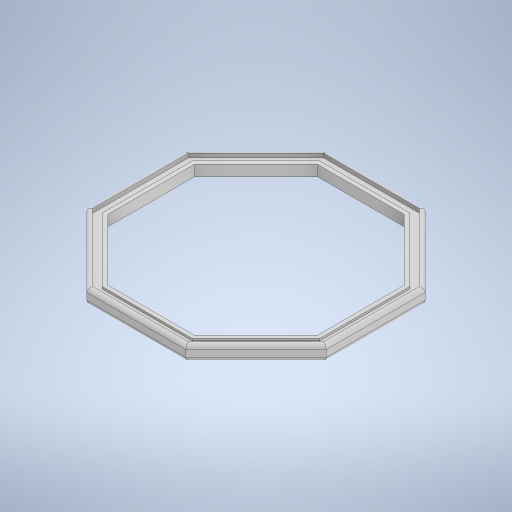
# Autodesk Inventor part: OV-PAM_ring_2
Saved by Autodesk Inventor 2024 (Build 280153000, 153)
## iProperties
Created: 2023-06-19
Part Number: OV-PAM_ring_2
Material: 일반
Document SubType Name: Modeling
Designer: jsw
Density: 1 g/cm^3
Appearance: 기본값
Author: jsw
Autodesk Inventor part; units mm, degrees
ref_plane "YZ Plane" through (0, 0, 0) normal (1, 0, 0) x (0, 1, 0)
sketch "스케치1" plane through (0, 0, 0) normal (0, 1, 0) x (-1, 0, 0)
  line L0 (-32.5919, 13.5) -> (-13.5, 32.5919)
  line L1 (-13.5, 32.5919) -> (13.5, 32.5919)
  line L2 (13.5, 32.5919) -> (32.5919, 13.5)
  line L3 (32.5919, 13.5) -> (32.5919, -13.5)
  line L4 (32.5919, -13.5) -> (13.5, -32.5919)
  line L5 (13.5, -32.5919) -> (-13.5, -32.5919)
  line L6 (-13.5, -32.5919) -> (-32.5919, -13.5)
  line L7 (-32.5919, -13.5) -> (-32.5919, 13.5)
  line L8 (35.5919, 14.7426) -> (35.5919, -14.7426)
  line L9 (35.5919, -14.7426) -> (14.7426, -35.5919)
  line L10 (14.7426, -35.5919) -> (-14.7426, -35.5919)
  line L11 (-14.7426, -35.5919) -> (-35.5919, -14.7426)
  line L12 (-35.5919, -14.7426) -> (-35.5919, 14.7426)
  line L13 (-35.5919, 14.7426) -> (-14.7426, 35.5919)
  line L14 (-14.7426, 35.5919) -> (14.7426, 35.5919)
  line L15 (14.7426, 35.5919) -> (35.5919, 14.7426)
  point P0 (0, 0)
  point P1 (0, 0)
  point P2 (0, 0)
  dimension "d0" = 27
  dimension "d1" = 3
  constraints: 32 end point, 2 coincident, 2 horizontal, 34 other
  measures "d0" distance of L2.end L3.end
  measures "d1" distance between parallel lines of L8 L3
extrude "돌출1" add sketch "스케치1" along normal blind 4.4 contours L0 L1 L2 L3 L4 L5 L6 L7 | L8 L9 L10 L11 L12 L13 L14 L15
sketch "스케치3" plane through (0, 0, 0) normal (0, -1, 0) x (1, 0, 0)
  line L0 (-13.5, 32.5919) -> (13.5, 32.5919)
  line L1 (13.5, 32.5919) -> (32.5919, 13.5)
  line L2 (32.5919, 13.5) -> (32.5919, -13.5)
  line L3 (32.5919, -13.5) -> (13.5, -32.5919)
  line L4 (13.5, -32.5919) -> (-13.5, -32.5919)
  line L5 (-13.5, -32.5919) -> (-32.5919, -13.5)
  line L6 (-32.5919, -13.5) -> (-32.5919, 13.5)
  line L7 (-32.5919, 13.5) -> (-13.5, 32.5919)
  line L8 (-14.2456, 34.3919) -> (14.2456, 34.3919)
  line L9 (14.2456, 34.3919) -> (34.3919, 14.2456)
  line L10 (34.3919, 14.2456) -> (34.3919, -14.2456)
  line L11 (34.3919, -14.2456) -> (14.2456, -34.3919)
  line L12 (14.2456, -34.3919) -> (-14.2456, -34.3919)
  line L13 (-14.2456, -34.3919) -> (-34.3919, -14.2456)
  line L14 (-34.3919, -14.2456) -> (-34.3919, 14.2456)
  line L15 (-34.3919, 14.2456) -> (-14.2456, 34.3919)
  line L16 (-13.4172, 32.3919) -> (13.4172, 32.3919)
  line L17 (13.4172, 32.3919) -> (32.3919, 13.4172)
  line L18 (32.3919, 13.4172) -> (32.3919, -13.4172)
  line L19 (32.3919, -13.4172) -> (13.4172, -32.3919)
  line L20 (13.4172, -32.3919) -> (-13.4172, -32.3919)
  line L21 (-13.4172, -32.3919) -> (-32.3919, -13.4172)
  line L22 (-32.3919, -13.4172) -> (-32.3919, 13.4172)
  line L23 (-32.3919, 13.4172) -> (-13.4172, 32.3919)
  point P0 (0, 0)
  point P1 (0, 0)
  point P2 (0, 0)
  point P3 (0, 0)
  dimension "d8" = 27
  dimension "d9" = 1.8
  dimension "d19" = 0.2
  constraints: 48 end point, 3 coincident, 3 horizontal, 51 other
  measures "d8" distance of L0.start L0.end
  measures "d9" distance between parallel lines of L8 L0
  measures "d19" distance between parallel lines of L16 L0
extrude "돌출3" cut sketch "스케치3" against normal blind 1.2 contours L0 L1 L2 L3 L4 L5 L6 L7 | L8 L9 L10 L11 L12 L13 L14 L15
ref_plane "작업 평면1" through (0, 2.4, 0) normal (0, 1, 0) x (1, 0, 0)
fillet "모깎기1" radius 1.2 16 edges at (-25.1673, 4.4, -25.1673) (-35.5919, 4.4, 0) (-25.1673, 4.4, 25.1673) (0, 4.4, 35.5919) (25.1673, 4.4, 25.1673) (35.5919, 4.4, 0) (25.1673, 4.4, -25.1673) (0, 4.4, -35.5919) (-25.1673, 0, 25.1673) (-35.5919, 0, 0) (-25.1673, 0, -25.1673) (0, 0, -35.5919) (25.1673, 0, -25.1673) (35.5919, 0, 0) (25.1673, 0, 25.1673) (0, 0, 35.5919)
sketch "스케치12" plane through (0, 0, 0) normal (0, -1, 0) x (1, 0, 0)
  line L0 (12.9201, -31.1919) -> (-12.9201, -31.1919)
  line L1 (-12.9201, -31.1919) -> (-31.1919, -12.9201)
  line L2 (-31.1919, -12.9201) -> (-31.1919, 12.9201)
  line L3 (-31.1919, 12.9201) -> (-12.9201, 31.1919)
  line L4 (-12.9201, 31.1919) -> (12.9201, 31.1919)
  line L5 (12.9201, 31.1919) -> (31.1919, 12.9201)
  line L6 (31.1919, 12.9201) -> (31.1919, -12.9201)
  line L7 (31.1919, -12.9201) -> (12.9201, -31.1919)
  line L8 (32.3919, -13.4172) -> (32.3919, 13.4172) projected
  point P0 (0, 0)
  point P1 (0, 0)
  dimension "d131" = 1.2
  constraints: 16 end point, 1 coincident, 1 horizontal, 17 other
  measures "d131" distance between parallel lines of L6 L8
extrude "돌출13" cut sketch "스케치12" against normal blind 10
sketch "스케치13" plane through (0, 0, 0) normal (0, -1, 0) x (1, 0, 0)
  line L0 (12.9201, 31.1919) -> (31.1919, 12.9201) projected
  line L1 (31.1919, 12.9201) -> (31.1919, -12.9201) projected
  line L2 (31.1919, -12.9201) -> (12.9201, -31.1919) projected
  line L3 (12.9201, -31.1919) -> (-12.9201, -31.1919) projected
  line L4 (-12.9201, -31.1919) -> (-31.1919, -12.9201) projected
  line L5 (-31.1919, -12.9201) -> (-31.1919, 12.9201) projected
  line L6 (-31.1919, 12.9201) -> (-12.9201, 31.1919) projected
  line L7 (-12.9201, 31.1919) -> (12.9201, 31.1919) projected
  line L8 (32.3919, 13.4172) -> (13.4172, 32.3919) projected
  line L9 (13.4172, 32.3919) -> (-13.4172, 32.3919) projected
  line L10 (-13.4172, 32.3919) -> (-32.3919, 13.4172) projected
  line L11 (-32.3919, 13.4172) -> (-32.3919, -13.4172) projected
  line L12 (-32.3919, -13.4172) -> (-13.4172, -32.3919) projected
  line L13 (-13.4172, -32.3919) -> (13.4172, -32.3919) projected
  line L14 (13.4172, -32.3919) -> (32.3919, -13.4172) projected
  line L15 (32.3919, -13.4172) -> (32.3919, 13.4172) projected
  point P0 (0, 0)
ref_plane "작업 평면2" through (0, 2.2, 0) normal (0, -1, 0) x (1, 0, 0)
extrude "돌출15" cut sketch "스케치13" against normal blind 0.6
mirror "미러5" about plane through (0, 2.2, 0) normal (0, -1, 0) of "돌출3", "돌출15"
